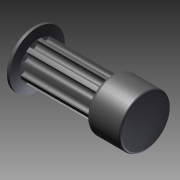
# Autodesk Inventor part: zrr_htd_3m15_0_17031000
Saved by Autodesk Inventor 2011 SP1 (Build 150282100, 282)
## iProperties
Created: 2018-07-07
Part Number: zrr_htd_3m15_0_17031000
Catalog Web Link: www.cadenas.de
Description: zrr_htd_3m15-HTD Pulleys Profile 3M, Timing Belt Width 15mm
Vendor: MAEDLER
Document SubType Name: Modeling
Designer: psAdmin
Manufacturer: MAEDLER
Mass: 5 g
Surface Area: 14.2236 cm^2
Volume: 1.71146 cm^3
Density: 1 g/cm^3
Category: PARTsolutions
Company: MAEDLER
Title: zrr_htd_3m15_0_17031000
Author: Cadenas PARTsolutions
Comments: HTD Pulleys Profile 3M, Timing Belt Width 15mm
PSOL_IDENT_0: {$CADENAS_DATA\23d-libs\maedler\antriebselemente\zahnriemenraeder_zahnriemen\zahnriemenraeder\htd-pr
PSOL_IDENT_1: ofil\zrr_htd_3m15.prj},197 {VTYP=3D},{NB=zrr_htd_3m15_0_17031000},{LINA=zrr_htd_3m15_0_17031000},{NN=
PSOL_IDENT_2: zrr_htd_3m15},{DATE=16.06.2017 10:47:49},{GEOMDATE=09.06.2016 09:07:07},{VERSION=},{LINEID=210},{LIN
PSOL_IDENT_3: ESUBID=-1},{WBVAR=BX}  {NB=zrr_htd_3m15_0_17031000},{LINA=zrr_htd_3m15_0_17031000},{KT=DUMMY},{ARTNR=
PSOL_IDENT_4: 17031000},{PDF=PDF Katalogseite},{AUSF=10-3M-15-0F},{MAT=Aluminium},{ZTL=3.000},{ZRB=15.000},{Z=10.0
PSOL_IDENT_5: 00},{AUS=0F},{ZS=8.790},{BS=13.000},{DO=9.550},{ND=12.000},{B=17.000},{L=26.000},{I=0.000},{VB=0.000
PSOL_IDENT_6: },{FB=3.500},{BX=0},{GEW=5.000},{ZT=1.200},{ZB=1.800},{T=0.000},{BB=1.000}
NN: zrr_htd_3m15
NT: HTD-Zahnriemenräder Profil 3M, Zahnriemenbreite 15mm
NB: zrr_htd_3m15_0_17031000
NBSYN: zrr_htd_3m15_$BX._$ARTNR.
LINA: zrr_htd_3m15_0_17031000
ARTNR: 17031000
PDF: PDF Katalogseite
AUSF: 10-3M-15-0F
MAT: Aluminium
ZTL: 3.000
ZRB: 15.000
Z: 10.000
AUS: 0F
ZS: 8.790
BS: 13.000
DO: 9.550
ND: 12.000
B: 17.000
L: 26.000
I: 0.000
VB: 0.000
FB: 3.500
BX: 0
GEW: 5.000
ZT: 1.200
ZB: 1.800
T: 0.000
BB: 1.000
SUPPLIER: MAEDLER
ARTICLENO: zrr_htd_3m15_0_17031000
BOMINFO: zrr_htd_3m15_0_17031000
CREATOR: CADENAS GmbH
Autodesk Inventor part; units mm, degrees
ref_plane "YZ Plane" through (0, 0, 0) normal (1, 0, 0) x (0, 1, 0)
ref_plane "XZ Plane" through (0, 0, 0) normal (0, 1, 0) x (-1, 0, 0)
ref_plane "XY Plane" through (0, 0, 0) normal (0, 0, 1) x (1, 0, 0)
sketch "Sketch_1" plane through (0, 0, 0) normal (0, 0, 1) x (1, 0, 0)
  line L0 (500, 0) -> (-500, 0)
  line L1 (0.3712, 0) -> (0.3712, 4.395)
  line L2 (0.3712, 4.395) -> (0, 6.5)
  line L3 (0, 6.5) -> (0.6288, 6.5)
  line L4 (0.6288, 6.5) -> (1, 4.395)
  line L5 (1, 4.395) -> (18, 4.395)
  line L6 (18, 4.395) -> (18, 5)
  arc A0 (19, 6) -> (18, 5) centre (19, 5) ccw
  line L7 (19, 6) -> (25.5, 6)
  arc A1 (26, 5.5) -> (25.5, 6) centre (25.5, 5.5) ccw
  line L8 (26, 5.5) -> (26, 0)
  line L9 (26, 0) -> (0.3712, 0)
  constraints: 20 end point, 4 point on circle, 2 centre point
revolve "Revolution1" add sketch "Sketch_1" angle 360 about axis through (500, 0, 0) along (1, 0, 0)
sketch "Sketch_2" plane through (1, 0, 0) normal (1, 0, 0) x (0, 0, -1)
  circle A0 centre (0, 0) radius 8.79
  arc A1 (-4.395, 0) -> (-4.3694, -0.4734) centre (0, 0) ccw
  line L0 (-4.3694, -0.4734) -> (-4.1727, -0.4095)
  arc A2 (-3.0386, -0.9873) -> (-4.1727, -0.4095) centre (-3.8946, -1.2654) ccw
  arc A3 (-3.6165, -2.1214) -> (-3.0386, -0.9873) centre (-3.8946, -1.2654) ccw
  line L1 (-3.6165, -2.1214) -> (-3.8132, -2.1853)
  arc A4 (-3.8132, -2.1853) -> (-3.5556, -2.5833) centre (0, 0) ccw
  arc A5 (-3.5556, -2.5833) -> (-3.2567, -2.9513) centre (0, 0) ccw
  line L2 (-3.2567, -2.9513) -> (-3.1351, -2.7839)
  arc A6 (-1.878, -2.5848) -> (-3.1351, -2.7839) centre (-2.407, -3.3129) ccw
  arc A7 (-1.6789, -3.8419) -> (-1.878, -2.5848) centre (-2.407, -3.3129) ccw
  line L3 (-1.6789, -3.8419) -> (-1.8005, -4.0093)
  arc A8 (-1.8005, -4.0093) -> (-1.3581, -4.1799) centre (0, 0) ccw
  arc A9 (-1.3581, -4.1799) -> (-0.9, -4.3019) centre (0, 0) ccw
  line L4 (-0.9, -4.3019) -> (-0.9, -4.095)
  arc A10 (0, -3.195) -> (-0.9, -4.095) centre (0, -4.095) ccw
  arc A11 (0.9, -4.095) -> (0, -3.195) centre (0, -4.095) ccw
  line L5 (0.9, -4.095) -> (0.9, -4.3019)
  arc A12 (0.9, -4.3019) -> (1.3581, -4.1799) centre (0, 0) ccw
  arc A13 (1.3581, -4.1799) -> (1.8005, -4.0093) centre (0, 0) ccw
  line L6 (1.8005, -4.0093) -> (1.6789, -3.8419)
  arc A14 (1.878, -2.5848) -> (1.6789, -3.8419) centre (2.407, -3.3129) ccw
  arc A15 (3.1351, -2.7839) -> (1.878, -2.5848) centre (2.407, -3.3129) ccw
  line L7 (3.1351, -2.7839) -> (3.2567, -2.9513)
  arc A16 (3.2567, -2.9513) -> (3.5556, -2.5833) centre (0, 0) ccw
  arc A17 (3.5556, -2.5833) -> (3.8132, -2.1853) centre (0, 0) ccw
  line L8 (3.8132, -2.1853) -> (3.6165, -2.1214)
  arc A18 (3.0386, -0.9873) -> (3.6165, -2.1214) centre (3.8946, -1.2654) ccw
  arc A19 (4.1727, -0.4095) -> (3.0386, -0.9873) centre (3.8946, -1.2654) ccw
  line L9 (4.1727, -0.4095) -> (4.3694, -0.4734)
  arc A20 (4.3694, -0.4734) -> (4.395, 0) centre (0, 0) ccw
  arc A21 (4.395, 0) -> (4.3694, 0.4734) centre (0, 0) ccw
  line L10 (4.3694, 0.4734) -> (4.1727, 0.4095)
  arc A22 (3.0386, 0.9873) -> (4.1727, 0.4095) centre (3.8946, 1.2654) ccw
  arc A23 (3.6165, 2.1214) -> (3.0386, 0.9873) centre (3.8946, 1.2654) ccw
  line L11 (3.6165, 2.1214) -> (3.8132, 2.1853)
  arc A24 (3.8132, 2.1853) -> (3.5556, 2.5833) centre (0, 0) ccw
  arc A25 (3.5556, 2.5833) -> (3.2567, 2.9513) centre (0, 0) ccw
  line L12 (3.2567, 2.9513) -> (3.1351, 2.7839)
  arc A26 (1.878, 2.5848) -> (3.1351, 2.7839) centre (2.407, 3.3129) ccw
  arc A27 (1.6789, 3.8419) -> (1.878, 2.5848) centre (2.407, 3.3129) ccw
  line L13 (1.6789, 3.8419) -> (1.8005, 4.0093)
  arc A28 (1.8005, 4.0093) -> (1.3581, 4.1799) centre (0, 0) ccw
  arc A29 (1.3581, 4.1799) -> (0.9, 4.3019) centre (0, 0) ccw
  line L14 (0.9, 4.3019) -> (0.9, 4.095)
  arc A30 (0, 3.195) -> (0.9, 4.095) centre (0, 4.095) ccw
  arc A31 (-0.9, 4.095) -> (0, 3.195) centre (0, 4.095) ccw
  line L15 (-0.9, 4.095) -> (-0.9, 4.3019)
  arc A32 (-0.9, 4.3019) -> (-1.3581, 4.1799) centre (0, 0) ccw
  arc A33 (-1.3581, 4.1799) -> (-1.8005, 4.0093) centre (0, 0) ccw
  line L16 (-1.8005, 4.0093) -> (-1.6789, 3.8419)
  arc A34 (-1.878, 2.5848) -> (-1.6789, 3.8419) centre (-2.407, 3.3129) ccw
  arc A35 (-3.1351, 2.7839) -> (-1.878, 2.5848) centre (-2.407, 3.3129) ccw
  line L17 (-3.1351, 2.7839) -> (-3.2567, 2.9513)
  arc A36 (-3.2567, 2.9513) -> (-3.5556, 2.5833) centre (0, 0) ccw
  arc A37 (-3.5556, 2.5833) -> (-3.8132, 2.1853) centre (0, 0) ccw
  line L18 (-3.8132, 2.1853) -> (-3.6165, 2.1214)
  arc A38 (-3.0386, 0.9873) -> (-3.6165, 2.1214) centre (-3.8946, 1.2654) ccw
  arc A39 (-4.1727, 0.4095) -> (-3.0386, 0.9873) centre (-3.8946, 1.2654) ccw
  line L19 (-4.1727, 0.4095) -> (-4.3694, 0.4734)
  arc A40 (-4.3694, 0.4734) -> (-4.395, 0) centre (0, 0) ccw
  constraints: 80 point on circle, 41 centre point, 40 end point
extrude "Extrusion1" cut sketch "Sketch_2" along normal blind 17
body "Solid1"
